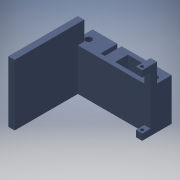
# Autodesk Inventor part: SupportPlateau
Saved by Autodesk Inventor 2017 SP1 (Build 210196100, 196)
## iProperties
Created: 2017-10-26
Part Number: SupportPlateau
Material: PC/ABS Plastic
Document SubType Name: Modeling
Designer: Biscuit
Density: 0.357273 g/cm^3
Appearance: Rubber - Blue
Author: Biscuit
Autodesk Inventor part; units mm, degrees
ref_plane "YZ Plane" through (0, 0, 0) normal (1, 0, 0) x (0, 1, 0)
ref_plane "XZ Plane" through (0, 0, 0) normal (0, 1, 0) x (-1, 0, 0)
ref_plane "XY Plane" through (0, 0, 0) normal (0, 0, 1) x (1, 0, 0)
sketch "Sketch3" plane through (0, 0, 0) normal (0, 0, 1) x (1, 0, 0)
  line L0 (0, 0) -> (75, 0)
  line L1 (75, 0) -> (75, 20)
  line L2 (75, 20) -> (0, 20)
  line L3 (0, 20) -> (0, 0)
  circle A0 centre (6.25, 10) radius 3
  circle A1 centre (68.75, 10) radius 3
  line L4 (37.5, 16) -> (57.5, 16)
  line L5 (57.5, 16) -> (57.5, 4)
  line L6 (57.5, 4) -> (37.5, 4)
  line L7 (37.5, 4) -> (37.5, 16)
  dimension "d19" = 20
  dimension "d20" = 75
  dimension "d21" = 6
  dimension "d22" = 6
  dimension "d23" = 10
  dimension "d24" = 10
  dimension "d25" = 62.5
  dimension "d26" = 6.25
  dimension "d30" = 12
  dimension "d31" = 20
  dimension "d32" = 4
  dimension "d33" = 17.5
  constraints: 16 end point, 4 parallel, 2 centre point, 2 horizontal, 2 perpendicular
  measures "d19" distance of L2.end L0.start
  measures "d20" distance of L1.end L2.end
  measures "d21" diameter of A0
  measures "d22" diameter of A1
  measures "d23" distance from line of L0 A0.centre
  measures "d24" distance from line of L0 A1.centre
  measures "d25" distance of A1.centre A0.centre
  measures "d26" distance from line of L3 A0.centre
  measures "d30" distance of L6.end L4.start
  measures "d31" distance of L4.start L4.end
  measures "d32" distance between parallel lines of L2 L4
  measures "d33" distance between parallel lines of L1 L5
extrude "Extrusion3" add sketch "Sketch3" along normal blind 40
sketch "Sketch4" plane through (0, 20, 0) normal (0, 1, 0) x (1, 0, 0)
  line L0 (0, 0) -> (75, 0) projected
  line L1 (27.5, -40) -> (27.5, -20)
  line L2 (27.5, -20) -> (15.5, -20)
  line L3 (15.5, -20) -> (15.5, -32)
  line L4 (15.5, -32) -> (23.5, -32)
  line L5 (23.5, -32) -> (23.5, -40)
  line L6 (17.5, -22) -> (25.5, -22)
  line L7 (25.5, -22) -> (25.5, -30)
  line L8 (25.5, -30) -> (17.5, -30)
  line L9 (17.5, -30) -> (17.5, -22)
  line L10 (23.5, -40) -> (27.5, -40)
  line L11 (0, 0) -> (0, -40) projected
  line L12 (75, -40) -> (0, -40) projected
  line L13 (75, 0) -> (75, -40) projected
  line L14 (27.5, 0) -> (27.5, -20)
  line L15 (15.5, -20) -> (15.5, -8)
  line L16 (15.5, -8) -> (23.5, -8)
  line L17 (23.5, -8) -> (23.5, 0)
  line L18 (17.5, -18) -> (25.5, -18)
  line L19 (25.5, -18) -> (25.5, -10)
  line L20 (25.5, -10) -> (17.5, -10)
  line L21 (17.5, -10) -> (17.5, -18)
  line L22 (23.5, 0) -> (27.5, 0)
  dimension "d34" = 2
  dimension "d35" = 2
  dimension "d36" = 2
  dimension "d37" = 2
  dimension "d38" = 4
  dimension "d39" = 32
  dimension "d40" = 8
  dimension "d41" = 8
  dimension "d42" = 27.5
  dimension "d43" = 40
  constraints: 38 end point, 8 symmetric about line, 5 perpendicular, 2 parallel
  measures "d34" distance between parallel lines of L1 L7
  measures "d35" distance between parallel lines of L3 L9
  measures "d36" distance between parallel lines of L2 L6
  measures "d37" distance between parallel lines of L4 L8
  measures "d38" distance between parallel lines of L1 L5
  measures "d39" distance between parallel lines of L0 L4
  measures "d40" distance between parallel lines of L7 L9
  measures "d41" distance between parallel lines of L8 L6
  measures "d42" distance between parallel lines of L11 L1
  measures "d43" distance between parallel lines of L0 L12
extrude "Extrusion4" cut sketch "Sketch4" against normal blind 16 contours L0 L14 L2 L15 L16 L17 | L5 L4 L3 L2 L1 L10
sketch "Sketch5" plane through (0, 0, 0) normal (0, -1, 0) x (1, 0, 0)
  line L0 (0, 0) -> (75, 0) projected
  line L1 (0, 40) -> (75, 40) projected
  line L2 (75, 0) -> (75, 40) projected
  line L3 (0, 0) -> (0, 40) projected
  line L4 (0, 40) -> (6, 40)
  line L5 (6, 40) -> (6, 58)
  line L6 (6, 58) -> (0, 58)
  line L7 (0, 58) -> (0, 40)
  line L8 (75, 40) -> (69, 40)
  line L9 (69, 40) -> (69, 58)
  line L10 (69, 58) -> (75, 58)
  line L11 (75, 58) -> (75, 40)
  dimension "d46" = 40
  dimension "d47" = 75
  dimension "d48" = 6
  dimension "d49" = 18
  dimension "d79" = 6
  dimension "d80" = 18
  constraints: 16 end point, 4 parallel, 2 horizontal, 2 perpendicular
  measures "d46" distance between parallel lines of L0 L1
  measures "d47" distance between parallel lines of L2 L3
  measures "d48" distance of L5.end L6.end
  measures "d49" distance of L6.end L1.start
  measures "d79" distance of L9.end L10.end
  measures "d80" distance of L8.end L9.end
extrude "Extrusion5" add sketch "Sketch5" against normal blind 6 contours L7 L6 L5 L1 | L1 L9 L10 L11
sketch "Esquisse12" plane through (75, 20, 40) normal (0, 1, 0) x (1, 0, 0)
  circle A0 centre (-15.75, 12) radius 1
  line L0 (-47.5, 40) -> (-47.5, 0)
  line L1 (0, 0) -> (-47.5, 0)
  line L2 (0, 40) -> (0, 0)
  line L3 (0, 40) -> (-47.5, 40)
  circle A1 centre (-31.75, 12) radius 1
  circle A2 centre (-15.75, 28) radius 1
  circle A3 centre (-31.75, 28) radius 1
  line L4 (0, 6) -> (0, 52)
  line L5 (0, 0) -> (63, 0)
  line L6 (0, 40) -> (0, 0) projected
  point P0 (-75, 40)
  point P1 (-6, 0)
  point P2 (-75, 40)
  point P3 (69, 26.5)
  point P4 (0, 52)
  dimension "d122" = 2
  dimension "d123" = 16
  dimension "d124" = 16
  dimension "d125" = 15.75
  dimension "d126" = 47.5
  dimension "d127" = 40
  dimension "d128" = 12
  dimension "d129" = 47.5
  constraints: 10 end point, 4 centre point, 2 collinear, 2 vertical, 1 horizontal, 9 other
  measures "d122" diameter of A0
  measures "d123" distance of A0.centre A1.centre
  measures "d124" distance of A0.centre A2.centre
  measures "d125" distance from line of L2 A0.centre
  measures "d126" distance of L1.start L0.end
  measures "d127" distance of L2.start L1.start
  measures "d128" distance from line of L1 A0.centre
  measures "d129" distance between parallel lines of L2 L0
extrude "Extrusion12" cut sketch "Esquisse12" against normal blind 5 contours A0 | A1 | A2 | A3
sketch "Esquisse13" plane through (0, 0, 0) normal (0, -1, 0) x (1, 0, 0)
  line L0 (0, 0) -> (0, 40) projected
  line L1 (0, 0) -> (6, 0)
  line L2 (6, 0) -> (6, 58)
  line L3 (6, 58) -> (0, 58)
  line L4 (0, 58) -> (0, 0)
  constraints: 8 end point, 2 parallel, 1 horizontal, 1 perpendicular
extrude "Extrusion13" add sketch "Esquisse13" along normal blind 60
sketch "Esquisse14" plane through (6, 0, 0) normal (0, -1, 0) x (1, 0, 0)
  line L0 (63, 58) -> (63, 40) projected
  line L1 (69, 0) -> (69, 58) projected
  line L2 (63, 58) -> (69, 58)
  line L3 (69, 58) -> (69, 52)
  line L4 (69, 52) -> (63, 52)
  line L5 (63, 52) -> (63, 58)
  line L6 (0, 0) -> (69, 0) projected
  line L7 (69, 0) -> (63, 0)
  line L8 (63, 0) -> (63, 6)
  line L9 (63, 6) -> (69, 6)
  line L10 (69, 6) -> (69, 0)
  point P0 (-6, 0)
  dimension "d134" = 6
  dimension "d135" = 6
  dimension "d136" = 6
  dimension "d137" = 6
  constraints: 16 end point, 4 parallel, 2 horizontal, 2 perpendicular, 1 point on line
  measures "d134" distance between parallel lines of L1 L0
  measures "d135" distance of L8.end L9.end
  measures "d136" distance between parallel lines of L2 L4
  measures "d137" distance between parallel lines of L6 L9
extrude "Extrusion14" add sketch "Esquisse14" along normal blind 8
sketch "Esquisse15" plane through (69, 6, 58) normal (0, 0, 1) x (1, 0, 0)
  circle A0 centre (3, -11) radius 1.5
  line L0 (6, -14) -> (0, -14) projected
  line L1 (-63, -6) -> (0, -6) projected
  line L2 (6, -6) -> (6, -14) projected
  point P0 (-69, -6)
  dimension "d140" = 3
  dimension "d141" = 3
  dimension "d142" = 6
  dimension "d143" = 8
  dimension "d144" = 3
  constraints: 1 centre point
  measures "d140" diameter of A0
  measures "d141" distance from line of L0 A0.centre
  measures "d142" distance of L0.start L0.end
  measures "d143" distance between parallel lines of L1 L0
  measures "d144" distance from line of L2 A0.centre
extrude "Extrusion15" cut sketch "Esquisse15" against normal through all
fillet "Congé2" radius 3 4 edges at (69, -8, 55) (75, -8, 55) (75, -8, 3) (69, -8, 3)
equation "\"d22\" = d21"
equation "\"d23\" = 0.5 * d19"
equation "\"d24\" = 0.5 * d19"
equation "\"d26\" = 0.5 * d20 - 0.5 * d25"
equation "\"d32\" = 0.5 * d19 - 0.5 * d30"
equation "\"d33\" = 0.5 * d20 - d31"
equation "\"d35\" = d34"
equation "\"d36\" = d34"
equation "\"d37\" = d34"
equation "\"d38\" = 2 * d34"
equation "\"d40\" = 4 * d34"
equation "\"d41\" = 4 * d34"
equation "\"d79\" = d48"
equation "\"d80\" = d49"
equation "\"d125\" = 0.5 * d126 - 0.5 * d123"
equation "\"d128\" = 0.5 * d127 - 0.5 * d124"
equation "\"d135\" = d134"
equation "\"d136\" = d134"
equation "\"d137\" = d136"
equation "\"d144\" = 0.5 * d142"
body "Solid2"
